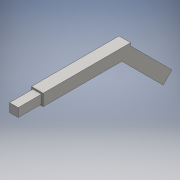
# Autodesk Inventor part: Stalk
Saved by Autodesk Inventor 2016 (Build 200138000, 138)
## iProperties
Created: 2015-09-21
Part Number: Stalk
Material: Generic
Document SubType Name: Modeling
Designer: Zachary
Density: 1 g/cm^3
Appearance: Default
Author: Zachary
Autodesk Inventor part; units mm, degrees
ref_plane "YZ Plane" through (0, 0, 0) normal (1, 0, 0) x (0, 1, 0)
ref_plane "XZ Plane" through (0, 0, 0) normal (0, 1, 0) x (-1, 0, 0)
ref_plane "XY Plane" through (0, 0, 0) normal (0, 0, 1) x (1, 0, 0)
sketch "Sketch1" plane through (0, 0, 0) normal (0, 1, 0) x (-1, 0, 0)
  line L0 (-2.95, 2.95) -> (2.95, 2.95)
  line L1 (2.95, 2.95) -> (2.95, -2.95)
  line L2 (2.95, -2.95) -> (-2.95, -2.95)
  line L3 (-2.95, -2.95) -> (-2.95, 2.95)
  line L4 (-2.95, 2.95) -> (2.95, -2.95) construction
  line L5 (2.95, 2.95) -> (-2.95, -2.95) construction
  point P0 (0, 0)
  dimension "d0" = 5.9
  dimension "d1" = 5.9
  constraints: 12 end point, 2 midpoint, 2 parallel, 1 horizontal, 1 perpendicular
  measures "d0" distance of L1.end L2.end
  measures "d1" distance of L0.end L1.end
extrude "Extrusion1" add sketch "Sketch1" along normal blind 16
sketch "Sketch2" plane through (0, 16, 0) normal (0, 1, 0) x (1, 0, 0)
  line L0 (4, -4) -> (-4, -4)
  line L1 (-4, -4) -> (-4, 4)
  line L2 (-4, 4) -> (4, 4)
  line L3 (4, 4) -> (4, -4)
  line L4 (4, -4) -> (-4, 4) construction
  line L5 (-4, -4) -> (4, 4) construction
  point P0 (0, 0)
  dimension "d4" = 8
  dimension "d5" = 8
  constraints: 12 end point, 2 midpoint, 2 parallel, 1 horizontal, 1 perpendicular
  measures "d4" distance of L1.end L2.end
  measures "d5" distance of L0.end L1.end
extrude "Extrusion2" add sketch "Sketch2" along normal blind 60
chamfer "Chamfer1" distance 6 angle 45 1 edges at (0, 76, -4) measured on face at (1.3333, 76, 1.3333)
sketch "Sketch4" plane through (4, 76, 2) normal (0, 0.7071, -0.7071) x (-1, 0, 0)
  line L0 (8, -8.4853) -> (8, 0) projected
  line L1 (8, 0) -> (0, 0) projected
  line L2 (0, 0) -> (0, -8.4853) projected
  line L3 (0, -8.4853) -> (8, -8.4853) projected
  point P0 (4, -55.1543)
extrude "Extrusion4" add sketch "Sketch4" along normal blind 40
sketch "Sketch5" plane through (4, 104.2843, -26.2843) normal (0, 0.7071, -0.7071) x (-1, 0, 0)
  line L0 (8, -8.4853) -> (8, 0) projected
  line L1 (8, 0) -> (0, 0) projected
  line L2 (0, 0) -> (0, -8.4853) projected
  line L3 (0, -8.4853) -> (8, -8.4853) projected
  line L4 (7, -7.2426) -> (1, -7.2426)
  line L5 (1, -7.2426) -> (1, -1.2426)
  line L6 (1, -1.2426) -> (7, -1.2426)
  line L7 (7, -1.2426) -> (7, -7.2426)
  line L8 (7, -7.2426) -> (1, -1.2426) construction
  line L9 (1, -7.2426) -> (7, -1.2426) construction
  point P0 (4, -55.1543)
  point P1 (4, -4.2426)
  dimension "d15" = 6
  dimension "d16" = 6
  constraints: 12 end point, 2 midpoint, 2 parallel, 1 horizontal, 1 perpendicular
  measures "d15" distance of L5.end L6.end
  measures "d16" distance of L4.end L5.end
extrude "Extrusion5" cut sketch "Sketch5" against normal blind 10 contours L4 L5 L6 L7
body "Solid1"
